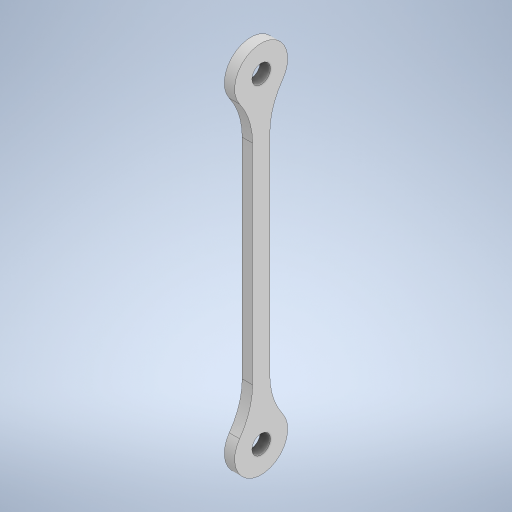
# Autodesk Inventor part: ön differansiyel
Saved by Autodesk Inventor 2023.2 (Build 272271000, 271)
## iProperties
Created: 2022-12-16
Part Number: ön differansiyel
Material: Generic
Document SubType Name: Modeling
Designer: omrfrkmll
Density: 1 g/cm^3
Appearance: Default
Author: omrfrkmll
Autodesk Inventor part; units mm, degrees
ref_plane "YZ Plane" through (0, 0, 0) normal (1, 0, 0) x (0, 1, 0)
ref_plane "XZ Plane" through (0, 0, 0) normal (0, 1, 0) x (-1, 0, 0)
ref_plane "XY Plane" through (0, 0, 0) normal (0, 0, 1) x (1, 0, 0)
sketch "Sketch1" plane through (0, 0, 0) normal (1, 0, 0) x (0, 1, 0)
  line L0 (0, 8.6387) -> (0, -8.0216)
  line L1 (-27.4792, 0) -> (24.1471, 0)
  circle A0 centre (-46.5, 0) radius 2.7
  circle A1 centre (46.5, 0) radius 2.7
  arc A2 (42.0088, -6.2545) -> (42.0088, 6.2545) centre (46.5, 0) ccw
  arc A3 (-42.0088, 6.2545) -> (-42.0088, -6.2545) centre (-46.5, 0) ccw
  line L2 (0, 2.5) -> (30.3433, 2.5)
  line L3 (0, 2.5) -> (-30.3433, 2.5)
  line L4 (0, -2.5) -> (-30.3433, -2.5)
  line L5 (0, -2.5) -> (30.3433, -2.5)
  arc A4 (30.3433, 2.5) -> (42.0088, 6.2545) centre (30.3433, 22.5) ccw
  arc A5 (42.0088, -6.2545) -> (30.3433, -2.5) centre (30.3433, -22.5) ccw
  arc A6 (-42.0088, 6.2545) -> (-30.3433, 2.5) centre (-30.3433, 22.5) ccw
  arc A7 (-30.3433, -2.5) -> (-42.0088, -6.2545) centre (-30.3433, -22.5) ccw
  point P0 (0, 0)
  point P1 (46.5, -7.7)
  point P2 (46.5, 7.7)
  point P3 (-46.5, -7.7)
  point P4 (-46.5, 7.7)
  point P5 (-39.2171, 2.5)
  point P6 (-39.2171, -2.5)
  point P7 (39.2171, -2.5)
  point P8 (39.2171, 2.5)
  dimension "d5" = 93
  dimension "d3" = 5
  dimension "d2" = 5
  dimension "d4" = 5.4
  dimension "d1" = 5
  dimension "d0" = 20
  constraints: 20 point on circle, 12 end point, 8 centre point, 8 tangent, 6 point on line, 4 equal radius, 4 horizontal, 4 symmetric about line, 2 vertical, 1 other
  measures "d5" distance of A1.centre A0.centre
  measures "d3" radial gap between concentric circles of A1 A2
  measures "d2" radial gap between concentric circles of A0 A3
  measures "d4" diameter of A1
  measures "d1" diameter of L2.start L1
  measures "d0" radius of A4
extrude "Extrusion1" add sketch "Sketch1" along normal blind 3
body "Solid1"
